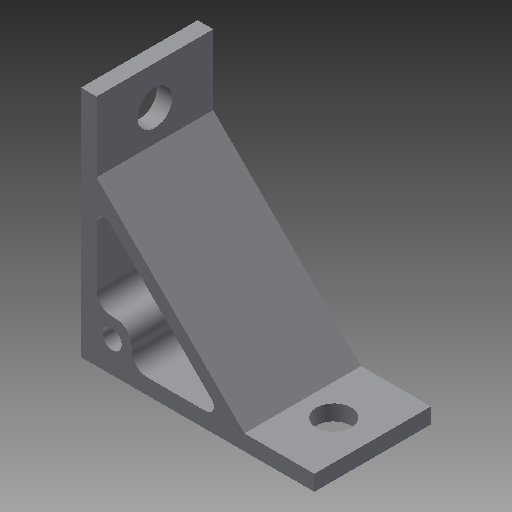
# Autodesk Inventor part: MayTec 1.46.20639_Angle Alu 60x60, D9.0, B30
Saved by Autodesk Inventor 2018 (Build 220112000, 112)
## iProperties
Category: PARTsolutions
Company: MAYTEC
Created: 2012-12-06
Part Number: MayTec 1.46.20639_Angle Alu 60x60, D9.0, B30
Catalog Web Link: www.cadenas.de
Description: Angles Alu-Angles Alu
Vendor: MAYTEC
Document SubType Name: Modeling
Designer: PARTuser1
Manufacturer: MAYTEC
Density: 1 g/cm^3
Material: Generic
Appearance: RGB(175.94999939203154,175.94999939203154,175.94999939203154)
PSOL_IDENT_0: {\\10.0.0.242\data_v9\23d-libs\maytec\maytec_3d\einbauzubehoer\winkel\winkel_alu\1.46.2.prj},234 {VT
PSOL_IDENT_1: YP=3D},{NB=MayTec 1.46.20639_Angle Alu 60x60, D9.0, B30},{LINA=MayTec 1.46.20639_Angle Alu 60x60, D9
PSOL_IDENT_2: .0, B30},{NN=Angles Alu},{DATE=14.09.2010 08:34:51},{GEOMDATE=28.01.2010 00:00:00},{VERSION=},{LINEI
PSOL_IDENT_3: D=50},{LINESUBID=-1},{WBVAR=}  {NB=MayTec 1.46.20639_Angle Alu 60x60, D9.0, B30},{LINA=MayTec 1.46.2
PSOL_IDENT_4: 0639_Angle Alu 60x60, D9.0, B30},{KT=DUMMY},{PARTNR=1.46.20639},{DESCRIPTION=Winkel Alu 60x60, D9.0,
PSOL_IDENT_5: B30},{L=60.000},{B=30.000},{WS=4.000},{BA1=8.000},{BA2=50.000},{BD=9.000},{NA=0.000},{NL=0.000},{LB
PSOL_IDENT_6: =42.000},{RB=2.000},{XTRANS=Angle Alu 60x60, D9.0, B30}
CNS_NT: Angles Alu
CNS_NB: MayTec 1.46.20639_Angle Alu 60x60, D9.0, B30
CNS_NBSYN: MayTec $PARTNR._$XTRANS.
CNS_LINA: MayTec 1.46.20639_Angle Alu 60x60, D9.0, B30
CNS_PARTNR: 1.46.20639
CNS_DESCRIPTION: Angle Alu 60x60, D9.0, B30
CNS_L: 60.000
CNS_B: 30.000
CNS_WS: 4.000
CNS_BA1: 8.000
CNS_BA2: 50.000
CNS_BD: 9.000
CNS_NA: 0.000
CNS_NL: 0.000
CNS_LB: 42.000
CNS_RB: 2.000
CNS_XTRANS: Angle Alu 60x60, D9.0, B30
SUPPLIER: MAYTEC
ARTICLENO: MayTec 1.46.20639_Angle Alu 60x60, D9.0, B30
BOMINFO: MayTec 1.46.20639_Angle Alu 60x60, D9.0, B30
CREATOR: CADENAS GmbH
Title: MayTec 1.46.20639_Angle Alu 60x60, D9.0, B30
Author: Cadenas PARTsolutions
Comments: Angles Alu
Autodesk Inventor part; units mm, degrees
sketch "Skizze_1" plane through (0, 0, 0) normal (0, 0, 1) x (1, 0, 0)
  line L0 (0, 0) -> (60, 0)
  line L1 (60, 0) -> (60, 4)
  line L2 (60, 4) -> (42, 4)
  line L3 (42, 4) -> (4, 42)
  line L4 (4, 42) -> (4, 60)
  line L5 (4, 60) -> (0, 60)
  line L6 (0, 60) -> (0, 0)
  constraints: 14 end point
extrude "Extrusion1" add sketch "Skizze_1" along normal mid plane 30
sketch "Skizze_2" plane through (0, 0, 0) normal (0, 0, 1) x (1, 0, 0)
  arc A0 (4, 17) -> (8, 13) centre (8, 17) ccw
  line L0 (8, 13) -> (9, 13)
  arc A1 (13, 9) -> (9, 13) centre (9, 9) ccw
  line L1 (13, 9) -> (13, 8)
  arc A2 (13, 8) -> (17, 4) centre (17, 8) ccw
  line L2 (17, 4) -> (32.1716, 4)
  arc A3 (32.1716, 4) -> (33.5858, 7.4142) centre (32.1716, 6) ccw
  line L3 (33.5858, 7.4142) -> (7.4142, 33.5858)
  arc A4 (7.4142, 33.5858) -> (4, 32.1716) centre (6, 32.1716) ccw
  line L4 (4, 32.1716) -> (4, 17)
  constraints: 10 end point, 10 point on circle, 5 centre point
extrude "Extrusion2" cut sketch "Skizze_2" along normal mid plane 32
sketch "Skizze_3" plane through (0, 0, 0) normal (0, 0, 1) x (1, 0, 0)
  circle A0 centre (8, 8) radius 2.5
  constraints: 1 centre point
extrude "Extrusion3" cut sketch "Skizze_3" along normal mid plane 32
sketch "Sketch4" plane through (0, 0, 15) normal (0, -1, 0) x (1, 0, 0)
  point P0 (50, -15)
hole "Drilling 2" at (50, 0, 0) direction (0, 1, 0) diameter 9 depth 5
sketch "Sketch5" plane through (0, 0, 15) normal (-1, 0, 0) x (0, 0, 1)
  point P0 (-15, 50)
hole "Drilling 3" at (0, 50, 0) direction (1, 0, 0) diameter 9 depth 5
ref_plane "cover_panel_hole_a_XY" through (8, 8, 15) normal (0, 0, 1) x (1, 0, 0)
ref_plane "cover_panel_hole_a_YZ" through (8, 8, 15) normal (1, 0, 0) x (0, 1, 0)
ref_plane "cover_panel_hole_a_ZX" through (8, 8, 15) normal (0, 1, 0) x (0, 0, 1)
ref_plane "cover_panel_hole_b_XY" through (8, 8, -15) normal (0, 0, -1) x (1, 0, 0)
ref_plane "cover_panel_hole_b_YZ" through (8, 8, -15) normal (1, 0, 0) x (0, -1, 0)
ref_plane "cover_panel_hole_b_ZX" through (8, 8, -15) normal (0, -1, 0) x (0, 0, -1)
ref_plane "side_1_XY" through (0, 30, 0) normal (-1, 0, 0) x (0, 0, 1)
ref_plane "side_1_YZ" through (0, 30, 0) normal (0, 0, 1) x (0, 1, 0)
ref_plane "side_1_ZX" through (0, 30, 0) normal (0, 1, 0) x (-1, 0, 0)
ref_plane "side_2_XY" through (30, 0, 0) normal (0, -1, 0) x (0, 0, 1)
ref_plane "side_2_YZ" through (30, 0, 0) normal (0, 0, 1) x (-1, 0, 0)
ref_plane "side_2_ZX" through (30, 0, 0) normal (-1, 0, 0) x (0, -1, 0)
body "Solid1"
